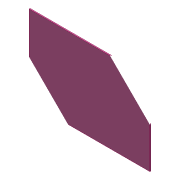
# Autodesk Inventor part: Starting position pink
Saved by Autodesk Inventor 2015 (Build 190159000, 159)
## iProperties
Created: 2015-03-07
Part Number: Starting position pink
Material: Generic
Document SubType Name: Modeling
Designer: Vukica
Density: 1 g/cm^3
Appearance: Default
Author: Vukica
Autodesk Inventor part; units mm, degrees
ref_plane "YZ Plane" through (0, 0, 0) normal (1, 0, 0) x (0, 1, 0)
ref_plane "XZ Plane" through (0, 0, 0) normal (0, 1, 0) x (-1, 0, 0)
ref_plane "XY Plane" through (0, 0, 0) normal (0, 0, 1) x (1, 0, 0)
sketch "Sketch1" plane through (0, 0, 0) normal (0, 0, 1) x (1, 0, 0)
  line L0 (0, 0) -> (762, 0)
  line L1 (762, 0) -> (762, 508)
  line L2 (762, 508) -> (0, 508)
  line L3 (0, 508) -> (0, 0)
  dimension "d0" = 762
  dimension "d1" = 508
  constraints: 8 end point, 2 parallel, 1 horizontal, 1 perpendicular
  measures "d0" distance of L1.end L2.end
  measures "d1" distance of L2.end L0.start
extrude "Extrusion1" add sketch "Sketch1" along normal blind 6.35
body "Solid1"
